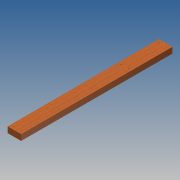
# Autodesk Inventor part: hubjig_cross
Saved by Autodesk Inventor 2014 SP1 (Build 180222100, 222)
## iProperties
Created: 2014-08-29
Part Number: hubjig_cross
Material: Wood (Cherry)
Document SubType Name: Modeling
Designer: Dave
Mass: 1951.21 g
Surface Area: 2390.32 cm^2
Volume: 3097.16 cm^3
Density: 0.63 g/cm^3
Appearance: Cherry - Natural Low Gloss
Author: Dave
Autodesk Inventor part; units mm, degrees
ref_plane "YZ Plane" through (0, 0, 0) normal (1, 0, 0) x (0, 1, 0)
ref_plane "XZ Plane" through (0, 0, 0) normal (0, 1, 0) x (-1, 0, 0)
ref_plane "XY Plane" through (0, 0, 0) normal (0, 0, 1) x (1, 0, 0)
sketch "Sketch1" plane through (0, 0, 0) normal (0, 0, 1) x (1, 0, 0)
  line L0 (0, 0) -> (88.9, 0)
  line L1 (88.9, 0) -> (88.9, 38.1)
  line L2 (88.9, 38.1) -> (0, 38.1)
  line L3 (0, 38.1) -> (0, 0)
  point P0 (0, 0)
  dimension "d0" = 88.9
  dimension "d1" = 38.1
  constraints: 8 end point, 2 parallel, 1 horizontal, 1 perpendicular
  measures "d0" distance of L0.start L0.end
  measures "d1" distance of L2.end L0.start
extrude "Extrusion1" add sketch "Sketch1" along normal blind 990.6
sketch "Sketch2" plane through (0, 38.1, 0) normal (0, 1, 0) x (1, 0, 0)
  line L0 (88.9, 0) -> (0, 0) projected
  line L1 (0, 0) -> (0, -990.6) projected
  circle A0 centre (19.05, -19.05) radius 13.4295
  circle A1 centre (69.85, -19.05) radius 13.4295
  circle A2 centre (19.05, -971.55) radius 13.4295
  circle A3 centre (69.85, -971.55) radius 13.4295
  dimension "d4" = 19.05
  dimension "d5" = 19.05
  dimension "d8" = 50.8
  dimension "d11" = 952.5
  constraints: 4 centre point, 1 horizontal, 1 vertical, 6 other
  measures "d4" distance from line of A0.centre L0
  measures "d5" distance from line of A0.centre L1
  measures "d8" distance of A0.centre A1.centre
  measures "d11" distance of A0.centre A2.centre
hole "Hole1" at (69.85, 38.1, 971.55) at (19.05, 38.1, 971.55) at (69.85, 38.1, 19.05) at (19.05, 38.1, 19.05) direction (0, -1, 0) diameter 5.1054 end through all clearance for "Flat Head Machine Screw (82)" size "#10" standard "Ansi Unified Screw Threads"
sketch "Sketch3" plane through (0, 38.1, 0) normal (0, 1, 0) x (1, 0, 0)
  line L0 (88.9, 0) -> (0, 0) projected
  line L1 (0, 0) -> (0, -990.6) projected
  line L2 (88.9, 0) -> (88.9, -990.6) projected
  line L3 (0, -495.3) -> (88.9, -495.3) construction
  circle A0 centre (19.05, -266.7) radius 9.489
  line L4 (50.8, -495.3) -> (139.7, -495.3) construction
  circle A1 centre (69.85, -266.7) radius 9.489
  circle A2 centre (19.05, -723.9) radius 9.489
  circle A3 centre (69.85, -723.9) radius 9.489
  dimension "d21" = 228.6
  dimension "d24" = 50.8
  constraints: 4 centre point, 4 end point, 2 midpoint, 2 symmetric about line, 1 horizontal, 7 other
  measures "d21" distance from line of L3 A0.centre
  measures "d24" distance of L3.start L4.start
hole "Hole2" at (19.05, 38.1, 723.9) at (69.85, 38.1, 723.9) at (19.05, 38.1, 266.7) at (69.85, 38.1, 266.7) direction (0, -1, 0) diameter 5.1054 end through all clearance for "Flat Head Machine Screw (82)" size "#10" standard "Ansi Unified Screw Threads"
sketch "Sketch4" plane through (0, 0, 0) normal (0, -1, 0) x (1, 0, 0)
  line L0 (0, 0) -> (88.9, 0) projected
  line L1 (88.9, 0) -> (88.9, 990.6) projected
  line L2 (0, 990.6) -> (88.9, 990.6) projected
  line L3 (0, 0) -> (0, 990.6) projected
  line L4 (0, 495.3) -> (88.9, 495.3) construction
  line L5 (44.45, 990.6) -> (44.45, 0) construction
  circle A0 centre (31.75, 704.85) radius 5.059
  circle A1 centre (57.15, 704.85) radius 5.059
  circle A2 centre (31.75, 285.75) radius 5.059
  circle A3 centre (57.15, 285.75) radius 5.059
  dimension "d36" = 209.55
  dimension "d37" = 12.7
  constraints: 4 centre point, 4 end point, 4 midpoint, 3 symmetric about line, 3 other
  measures "d36" distance from line of L4 A0.centre
  measures "d37" distance from line of A0.centre L5
hole "Hole3" at (31.75, 0, 704.85) at (57.15, 0, 704.85) at (31.75, 0, 285.75) at (57.15, 0, 285.75) direction (0, 1, 0) diameter 5.1054 depth 25.4 tip angle 118 clearance for "Flat Head Machine Screw (82)" size "#10" standard "Ansi Unified Screw Threads"
body "Solid1"
